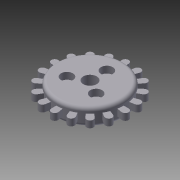
# Autodesk Inventor part: sprocket
Saved by Autodesk Inventor 2011 (Build 150239000, 239)
## iProperties
Created: 2010-04-19
Part Number: sprocket
Document SubType Name: Modeling
Designer: lucio
Density: 2.71 g/cm^3
Material: Aluminum-6061
Mass: 33.7054 g
Surface Area: 53.9873 cm^2
Volume: 12.4374 cm^3
Author: lucio
Autodesk Inventor part; units mm, degrees
ref_plane "YZ Plane" through (0, 0, 0) normal (1, 0, 0) x (0, 1, 0)
ref_plane "XZ Plane" through (0, 0, 0) normal (0, 1, 0) x (-1, 0, 0)
ref_plane "XY Plane" through (0, 0, 0) normal (0, 0, 1) x (1, 0, 0)
sketch "Sketch1" plane through (0, 0, 0) normal (0, 0, 1) x (1, 0, 0)
  arc A0 (0, 25) -> (-4.3412, 24.6202) centre (0, 0) ccw
  line L0 (0, 0) -> (-4.3412, 24.6202) construction
  line L1 (0, 0) -> (0, 25) construction
  line L2 (0, 25) -> (0, 0)
  line L3 (0, 0) -> (-4.3412, 24.6202)
  arc A1 (-8.5505, 23.4923) -> (-12.5, 21.6506) centre (0, 0) ccw
  line L4 (0, 0) -> (-12.5, 21.6506) construction
  line L5 (0, 0) -> (-8.5505, 23.4923) construction
  line L6 (-8.5505, 23.4923) -> (0, 0)
  line L7 (0, 0) -> (-12.5, 21.6506)
  arc A2 (-16.0697, 19.1511) -> (-19.1511, 16.0697) centre (0, 0) ccw
  line L8 (0, 0) -> (-19.1511, 16.0697) construction
  line L9 (0, 0) -> (-16.0697, 19.1511) construction
  line L10 (-16.0697, 19.1511) -> (0, 0)
  line L11 (0, 0) -> (-19.1511, 16.0697)
  arc A3 (-21.6506, 12.5) -> (-23.4923, 8.5505) centre (0, 0) ccw
  line L12 (0, 0) -> (-23.4923, 8.5505) construction
  line L13 (0, 0) -> (-21.6506, 12.5) construction
  line L14 (-21.6506, 12.5) -> (0, 0)
  line L15 (0, 0) -> (-23.4923, 8.5505)
  arc A4 (-24.6202, 4.3412) -> (-25, 0) centre (0, 0) ccw
  line L16 (0, 0) -> (-25, 0) construction
  line L17 (0, 0) -> (-24.6202, 4.3412) construction
  line L18 (-24.6202, 4.3412) -> (0, 0)
  line L19 (0, 0) -> (-25, 0)
  arc A5 (-24.6202, -4.3412) -> (-23.4923, -8.5505) centre (0, 0) ccw
  line L20 (0, 0) -> (-23.4923, -8.5505) construction
  line L21 (0, 0) -> (-24.6202, -4.3412) construction
  line L22 (-24.6202, -4.3412) -> (0, 0)
  line L23 (0, 0) -> (-23.4923, -8.5505)
  arc A6 (-21.6506, -12.5) -> (-19.1511, -16.0697) centre (0, 0) ccw
  line L24 (0, 0) -> (-19.1511, -16.0697) construction
  line L25 (0, 0) -> (-21.6506, -12.5) construction
  line L26 (-21.6506, -12.5) -> (0, 0)
  line L27 (0, 0) -> (-19.1511, -16.0697)
  arc A7 (-16.0697, -19.1511) -> (-12.5, -21.6506) centre (0, 0) ccw
  line L28 (0, 0) -> (-12.5, -21.6506) construction
  line L29 (0, 0) -> (-16.0697, -19.1511) construction
  line L30 (-16.0697, -19.1511) -> (0, 0)
  line L31 (0, 0) -> (-12.5, -21.6506)
  arc A8 (-8.5505, -23.4923) -> (-4.3412, -24.6202) centre (0, 0) ccw
  line L32 (0, 0) -> (-4.3412, -24.6202) construction
  line L33 (0, 0) -> (-8.5505, -23.4923) construction
  line L34 (-8.5505, -23.4923) -> (0, 0)
  line L35 (0, 0) -> (-4.3412, -24.6202)
  arc A9 (0, -25) -> (4.3412, -24.6202) centre (0, 0) ccw
  line L36 (0, 0) -> (4.3412, -24.6202) construction
  line L37 (0, 0) -> (0, -25) construction
  line L38 (0, -25) -> (0, 0)
  line L39 (0, 0) -> (4.3412, -24.6202)
  arc A10 (8.5505, -23.4923) -> (12.5, -21.6506) centre (0, 0) ccw
  line L40 (0, 0) -> (12.5, -21.6506) construction
  line L41 (0, 0) -> (8.5505, -23.4923) construction
  line L42 (8.5505, -23.4923) -> (0, 0)
  line L43 (0, 0) -> (12.5, -21.6506)
  arc A11 (16.0697, -19.1511) -> (19.1511, -16.0697) centre (0, 0) ccw
  line L44 (0, 0) -> (19.1511, -16.0697) construction
  line L45 (0, 0) -> (16.0697, -19.1511) construction
  line L46 (16.0697, -19.1511) -> (0, 0)
  line L47 (0, 0) -> (19.1511, -16.0697)
  arc A12 (21.6506, -12.5) -> (23.4923, -8.5505) centre (0, 0) ccw
  line L48 (0, 0) -> (23.4923, -8.5505) construction
  line L49 (0, 0) -> (21.6506, -12.5) construction
  line L50 (21.6506, -12.5) -> (0, 0)
  line L51 (0, 0) -> (23.4923, -8.5505)
  arc A13 (24.6202, -4.3412) -> (25, 0) centre (0, 0) ccw
  line L52 (0, 0) -> (25, 0) construction
  line L53 (0, 0) -> (24.6202, -4.3412) construction
  line L54 (24.6202, -4.3412) -> (0, 0)
  line L55 (0, 0) -> (25, 0)
  arc A14 (24.6202, 4.3412) -> (23.4923, 8.5505) centre (0, 0) ccw
  line L56 (0, 0) -> (23.4923, 8.5505) construction
  line L57 (0, 0) -> (24.6202, 4.3412) construction
  line L58 (24.6202, 4.3412) -> (0, 0)
  line L59 (0, 0) -> (23.4923, 8.5505)
  arc A15 (21.6506, 12.5) -> (19.1511, 16.0697) centre (0, 0) ccw
  line L60 (0, 0) -> (19.1511, 16.0697) construction
  line L61 (0, 0) -> (21.6506, 12.5) construction
  line L62 (21.6506, 12.5) -> (0, 0)
  line L63 (0, 0) -> (19.1511, 16.0697)
  arc A16 (16.0697, 19.1511) -> (12.5, 21.6506) centre (0, 0) ccw
  line L64 (0, 0) -> (12.5, 21.6506) construction
  line L65 (0, 0) -> (16.0697, 19.1511) construction
  line L66 (16.0697, 19.1511) -> (0, 0)
  line L67 (0, 0) -> (12.5, 21.6506)
  arc A17 (8.5505, 23.4923) -> (4.3412, 24.6202) centre (0, 0) ccw
  line L68 (0, 0) -> (4.3412, 24.6202) construction
  line L69 (0, 0) -> (8.5505, 23.4923) construction
  line L70 (8.5505, 23.4923) -> (0, 0)
  line L71 (0, 0) -> (4.3412, 24.6202)
  circle A18 centre (0, 0) radius 20
  dimension "d0" = 25
  dimension "d1" = 10
  dimension "d4" = 360
  dimension "d6" = 40
  constraints: 144 end point, 36 point on circle, 21 coincident, 19 centre point, 2 collinear, 161 other
  measures "d0" radius of A0
  measures "d1" angle of L1 L0
  measures "d6" diameter of A18
extrude "Extrusion1" add sketch "Sketch1" along normal mid plane 10 contours A18 L71 L2 | L2 L3 A18 | L3 L6 A18 | L7 A18 L6 | L10 A18 L7 | L11 A18 L10 | L14 A18 L11 | L15 A18 L14 | L18 A18 L15 | L19 A18 L18 | L22 A18 L19 | L23 A18 L22 | L26 A18 L23 | L27 A18 L26 | L30 A18 L27 | L31 A18 L30 | L34 A18 L31 | L35 A18 L34 | L38 A18 L35 | L39 A18 L38 | L42 A18 L39 | L43 A18 L42 | L46 A18 L43 | L47 A18 L46 | L50 A18 L47 | L51 A18 L50 | L54 A18 L51 | L55 A18 L54 | L58 A18 L55 | L59 A18 L58 | L62 A18 L59 | L63 A18 L62 | L66 A18 L63 | L67 A18 L66 | L70 A18 L67 | L71 A18 L70
extrude "Extrusion2" add sketch "Sketch1" along normal mid plane 4 contours L2 A18 L3 A0 | L2 L3 A18 | L7 A18 L6 | L11 A18 L10 | L15 A18 L14 | L19 A18 L18 | L23 A18 L22 | L27 A18 L26 | L31 A18 L30 | L35 A18 L34 | L39 A18 L38 | L43 A18 L42 | L47 A18 L46 | L51 A18 L50 | L55 A18 L54 | L59 A18 L58 | L63 A18 L62 | L67 A18 L66 | L71 A18 L70 | L71 A17 L70 A18 | A18 L7 A1 L6 | A18 L11 A2 L10 | A18 L15 A3 L14 | A18 L19 A4 L18 | A18 L23 A5 L22 | A18 L27 A6 L26 | A18 L31 A7 L30 | A18 L35 A8 L34 | A18 L39 A9 L38 | A18 L43 A10 L42 | A18 L47 A11 L46 | A18 L51 A12 L50 | A18 L55 A13 L54 | A18 L59 A14 L58 | A18 L63 A15 L62 | A18 L67 A16 L66
hole "Hole1" at (0, 0, 5) direction (0, 0, -1) diameter 8 end through all
fillet "Fillet1" radius 2 1 edges at (-20, 0, 5)
fillet "Fillet2" radius 2 36 edges at (-4.3412, -24.6202, 0) (-8.5505, -23.4923, 0) (0, -25, 0) (4.3412, -24.6202, 0) (8.5505, -23.4923, 0) (12.5, -21.6506, 0) (16.0697, -19.1511, 0) (19.1511, -16.0697, 0) (21.6506, -12.5, 0) (23.4923, -8.5505, 0) (24.6202, -4.3412, 0) (25, 0, 0) (24.6202, 4.3412, 0) (23.4923, 8.5505, 0) (21.6506, 12.5, 0) (19.1511, 16.0697, 0) (16.0697, 19.1511, 0) (12.5, 21.6506, 0) (8.5505, 23.4923, 0) (4.3412, 24.6202, 0) (0, 25, 0) (-4.3412, 24.6202, 0) (-8.5505, 23.4923, 0) (-12.5, 21.6506, 0) (-16.0697, 19.1511, 0) (-19.1511, 16.0697, 0) (-21.6506, 12.5, 0) (-23.4923, 8.5505, 0) (-24.6202, 4.3412, 0) (-25, 0, 0) (-24.6202, -4.3412, 0) (-23.4923, -8.5505, 0) (-21.6506, -12.5, 0) (-19.1511, -16.0697, 0) (-16.0697, -19.1511, 0) (-12.5, -21.6506, 0)
sketch "Sketch2" plane through (0, 0, 5) normal (0, 0, 1) x (1, 0, 0)
  circle A0 centre (0, 0) radius 4 projected
  point P0 (0, 10)
  point P1 (-8.6603, -5)
  point P2 (8.6603, -5)
  dimension "d22" = 10
  dimension "d25" = 360
  constraints: 4 other
  measures "d22" distance of A0.centre point (0, 10)
hole "Hole2" at (0, 10, 5) at (-8.6603, -5, 5) at (8.6603, -5, 5) direction (0, 0, -1) diameter 4 end through all counterbore diameter 7 counterbore depth 4
fillet "Fillet3" radius 2 1 edges at (-20, 0, -5)
body "Solid1"
